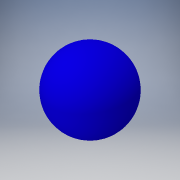
# Autodesk Inventor part: earth
Saved by Autodesk Inventor 2019 (Build 230136000, 136)
## iProperties
Created: 2019-09-02
Part Number: earth
Material: Generic
Document SubType Name: Modeling
Designer: james
Density: 1 g/cm^3
Appearance: Default
Author: james
Autodesk Inventor part; units mm, degrees
ref_plane "YZ Plane" through (0, 0, 0) normal (1, 0, 0) x (0, 1, 0)
ref_plane "XZ Plane" through (0, 0, 0) normal (0, 1, 0) x (-1, 0, 0)
ref_plane "XY Plane" through (0, 0, 0) normal (0, 0, 1) x (1, 0, 0)
sketch "Sketch1" plane through (0, 0, 0) normal (1, 0, 0) x (0, 1, 0)
  arc A0 (100552.2492, 12.7) -> (100552.2492, -12.7) centre (0, 0) ccw
  line L0 (100552.25, 0) -> (-100552.25, 0)
  line L1 (100577.65, 12.7) -> (100577.65, -12.7)
  line L2 (100552.2492, -12.7) -> (100577.65, -12.7)
  line L3 (100552.25, 0) -> (100577.65, 0)
  line L4 (100577.65, 12.7) -> (100552.2492, 12.7)
  dimension "d1" = 201104.5
  dimension "d9" = 90
  constraints: 10 end point, 3 point on circle, 1 centre point, 1 coincident, 1 horizontal, 1 midpoint
  measures "d1" diameter of A0
  measures "d9" angle of L4 L1
revolve "Revolution1" add sketch "Sketch1" angle 360 about axis through (0, 100552.25, 0) along (0, -1, 0) contours L4 L1 L3 L0 A0
sketch "Sketch2" plane through (0, 100577.65, 0) normal (0, 1, 0) x (1, 0, 0)
  circle A0 centre (0, 0) radius 190.5
  dimension "d11" = 381
  constraints: 1 centre point, 1 coincident
  measures "d11" diameter of A0
extrude "Extrusion1" add sketch "Sketch2" against normal blind 25.4
body "Solid1"
